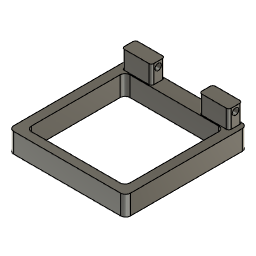
Korry_Protected_Base (Autodesk Fusion 360 design; units mm, degrees)
Autodesk Fusion 360 part; units mm, degrees
note: some values were not read from the file. Chosen so that the rebuilt part matches the saved one: which face or edge a step refers to. Set by a fixed rule: which sketch regions a step uses.
sketch "Sketch1" plane through (0, 0, 0) normal (0, 0, 1) x (1, 0, 0)
  line L0 (1, 0) -> (22.7, 0)
  line L1 (23.7, 1) -> (23.7, 23.7)
  line L2 (22.7, 24.7) -> (1, 24.7)
  line L3 (0, 23.7) -> (0, 1)
  line L4 (2.85, 21.75) -> (20.85, 21.75)
  line L5 (21.85, 20.75) -> (21.85, 2.75)
  line L6 (20.85, 1.75) -> (2.85, 1.75)
  line L7 (1.85, 2.75) -> (1.85, 20.75)
  arc A0 (2.85, 21.75) -> (1.85, 20.75) centre (2.85, 20.75) ccw
  arc A1 (1.85, 2.75) -> (2.85, 1.75) centre (2.85, 2.75) ccw
  arc A2 (21.85, 20.75) -> (20.85, 21.75) centre (20.85, 20.75) ccw
  arc A3 (20.85, 1.75) -> (21.85, 2.75) centre (20.85, 2.75) ccw
  arc A4 (1, 24.7) -> (0, 23.7) centre (1, 23.7) ccw
  arc A5 (22.7, 0) -> (23.7, 1) centre (22.7, 1) ccw
  arc A6 (0, 1) -> (1, 0) centre (1, 1) ccw
  arc A7 (23.7, 23.7) -> (22.7, 24.7) centre (22.7, 23.7) ccw
  point P0 (23.7, 0)
  point P1 (0, 24.7)
  point P2 (1.85, 21.75)
  point P3 (21.85, 21.75)
  point P4 (1.85, 1.75)
  dimension "d1" = 23.7
  dimension "d2" = 24.7
  dimension "d3" = 20
  dimension "d4" = 20
  dimension "d6" = 1.75
  dimension "d40" = 1.85
  dimension "d63" = 1
  dimension "d64" = 1
  dimension "d65" = 1
  dimension "d66" = 1
  dimension "d67" = 1
  dimension "d68" = 1
  dimension "d69" = 1
  dimension "d70" = 1
  constraint horizontal L0
  constraint vertical L1
  constraint horizontal L2
  constraint vertical L3
  constraint horizontal L4
  constraint vertical L5
  constraint horizontal L6
  constraint vertical L7
  constraint coincident P2 L4
  constraint coincident P2 L7
  constraint tangent L4 A0
  constraint tangent L7 A0
  constraint coincident P4 L6
  constraint coincident P4 L7
  constraint tangent L6 A1
  constraint tangent L7 A1
  constraint coincident P3 L4
  constraint coincident P3 L5
  constraint tangent L4 A2
  constraint tangent L5 A2
  constraint tangent L5 A3
  constraint tangent L6 A3
  constraint coincident P1 L2
  constraint coincident P1 L3
  constraint tangent L2 A4
  constraint tangent L3 A4
  constraint coincident P0 L0
  constraint coincident P0 L1
  constraint tangent L0 A5
  constraint tangent L1 A5
  constraint coincident origin L0
  constraint coincident origin L3
  constraint tangent L0 A6
  constraint tangent L3 A6
  constraint tangent L2 A7
  constraint tangent L1 A7
  measures "d1" distance of origin P0
  measures "d2" distance of origin P1
  measures "d3" distance of P2 P3
  measures "d4" distance of P2 P4
  measures "d6" distance of L0 L6
  measures "d40" distance of L3 L7
  measures "d63" radius of A0
  measures "d64" radius of A1
  measures "d65" radius of A2
  measures "d66" radius of A3
  measures "d67" radius of A4
  measures "d68" radius of A5
  measures "d69" radius of A6
  measures "d70" radius of A7
extrude "Extrude1" add sketch "Sketch1" along normal blind 4
sketch "Sketch2" plane through (0, 0, 4) normal (0, 0, 1) x (-1, 0, 0)
  line L0 (-20.85, -1.75) -> (-2.85, -1.75)
  line L1 (-1.85, -2.75) -> (-1.85, -20.75)
  line L2 (-2.85, -21.75) -> (-20.85, -21.75)
  line L3 (-21.85, -20.75) -> (-21.85, -2.75)
  line L4 (0, -23.7) -> (0, -1)
  line L5 (-1, 0) -> (-22.7, 0)
  line L6 (-23.7, -1) -> (-23.7, -23.7)
  line L7 (-22.7, -24.7) -> (-1, -24.7)
  line L8 (-1.5, -24.7) -> (-6.5, -24.7)
  line L9 (-7, -24.2) -> (-7, -22.45)
  line L10 (-6.5, -21.95) -> (-1.5, -21.95)
  line L11 (-1, -22.45) -> (-1, -24.2)
  line L12 (-22.2, -24.7) -> (-17.2, -24.7)
  line L13 (-16.7, -24.2) -> (-16.7, -22.45)
  line L14 (-17.2, -21.95) -> (-22.2, -21.95)
  line L15 (-22.7, -22.45) -> (-22.7, -24.2)
  arc A0 (-7, -24.2) -> (-6.5, -24.7) centre (-6.5, -24.2) ccw
  arc A1 (-6.5, -21.95) -> (-7, -22.45) centre (-6.5, -22.45) ccw
  arc A2 (-17.2, -24.7) -> (-16.7, -24.2) centre (-17.2, -24.2) ccw
  arc A3 (-16.7, -22.45) -> (-17.2, -21.95) centre (-17.2, -22.45) ccw
  arc A4 (-1.85, -2.75) -> (-2.85, -1.75) centre (-2.85, -2.75) ccw
  arc A5 (-2.85, -21.75) -> (-1.85, -20.75) centre (-2.85, -20.75) ccw
  arc A6 (-21.85, -20.75) -> (-20.85, -21.75) centre (-20.85, -20.75) ccw
  arc A7 (-20.85, -1.75) -> (-21.85, -2.75) centre (-20.85, -2.75) ccw
  arc A8 (0, -1) -> (-1, 0) centre (-1, -1) ccw
  arc A9 (-22.7, 0) -> (-23.7, -1) centre (-22.7, -1) ccw
  arc A10 (-1, -24.7) -> (0, -23.7) centre (-1, -23.7) ccw
  arc A11 (-23.7, -23.7) -> (-22.7, -24.7) centre (-22.7, -23.7) ccw
  arc A12 (-1, -22.45) -> (-1.5, -21.95) centre (-1.5, -22.45) ccw
  arc A13 (-1.5, -24.7) -> (-1, -24.2) centre (-1.5, -24.2) ccw
  arc A14 (-22.7, -24.2) -> (-22.2, -24.7) centre (-22.2, -24.2) ccw
  arc A15 (-22.2, -21.95) -> (-22.7, -22.45) centre (-22.2, -22.45) ccw
  point P0 (-1, -24.7)
  point P1 (-7, -24.7)
  point P2 (-22.7, -24.7)
  point P3 (-16.7, -24.7)
  dimension "d49" = 6
  dimension "d50" = 6
  dimension "d51" = 0.5
  dimension "d52" = 0.5
  dimension "d53" = 0.5
  dimension "d54" = 0.5
  dimension "d76" = 0.5
  dimension "d77" = 0.5
  dimension "d78" = 0.5
  dimension "d79" = 0.5
  constraint horizontal L8
  constraint vertical L9
  constraint horizontal L10
  constraint vertical L11
  constraint coincident P0 L7.end
  constraint horizontal L12
  constraint vertical L13
  constraint horizontal L14
  constraint vertical L15
  constraint coincident P2 L7.start
  constraint coincident P1 L8
  constraint coincident P1 L9
  constraint tangent L8 A0
  constraint tangent L9 A0
  constraint tangent L9 A1
  constraint tangent L10 A1
  constraint coincident P3 L12
  constraint coincident P3 L13
  constraint tangent L12 A2
  constraint tangent L13 A2
  constraint tangent L13 A3
  constraint tangent L14 A3
  constraint tangent L10 A12
  constraint tangent L11 A12
  constraint coincident P0 L11
  constraint coincident P0 L8
  constraint tangent L11 A13
  constraint tangent L8 A13
  constraint coincident P2 L12
  constraint coincident P2 L15
  constraint tangent L12 A14
  constraint tangent L15 A14
  constraint tangent L14 A15
  constraint tangent L15 A15
  measures "d49" distance of P0 P1
  measures "d50" distance of P2 P3
  measures "d51" radius of A0
  measures "d52" radius of A1
  measures "d53" radius of A2
  measures "d54" radius of A3
  measures "d76" radius of A12
  measures "d77" radius of A13
  measures "d78" radius of A14
  measures "d79" radius of A15
extrude "Extrude7" add sketch "Sketch2" along normal blind 5 contours L7 L8 L9 L10 L11 A0 A1 A12 A13 | L7 L12 L13 L14 L15 A2 A3 A14 A15
sketch "Sketch6" plane through (22.7, 0, 0) normal (1, 0, 0) x (0, 1, 0)
  line L0 (24.2, 9) -> (21.95, 9)
  line L1 (21.95, 9) -> (21.95, 4)
  line L2 (21.95, 4) -> (24.2, 4)
  line L3 (21.95, 4) -> (24.2, 9) construction
  line L4 (21.95, 9) -> (24.7, 4.3362) construction
  circle A0 centre (23.325, 6.6681) radius 0.65
  line L5 (24.2, 4) -> (24.2, 9)
  line L6 (22.45, 4) -> (24.2, 4)
  line L7 (24.2, 4) -> (24.2, 9)
  line L8 (24.2, 9) -> (22.45, 9)
  line L9 (22.45, 9) -> (22.45, 4)
  dimension "d57" = 1.3
  dimension "d80" = 2.3319
  constraint coincident L1.end L2.start
  constraint coincident L0.start L3.end
  constraint coincident L0.end L1.start
  constraint midpoint L4 A0.centre
  measures "d57" diameter of A0
  measures "d80" distance of L0 A0.centre
extrude "Extrude13" cut sketch "Sketch6" against normal blind 30 contours A0
extrude "Extrude12" cut 2 faces at (18.8667, 23.7833, 9) (3.1667, 23.7833, 9) along direction (0, 0, -1) blind 1.3
extrude "Extrude10" [suppressed]
extrude "Extrude8" [suppressed]
sketch "Sketch8" plane through (1, 0, 0) normal (-1, 0, 0) x (0, -1, 0)
  line L0 (-24.2, 4) -> (-22.45, 4)
  line L1 (-22.45, 9) -> (-24.2, 9)
  line L2 (-22.45, 9) -> (-24.2, 4) construction
  line L3 (-22.45, 4) -> (-24.2, 9) construction
  circle A0 centre (-23.325, 6.5) radius 0.65
  line L4 (-22.45, 4) -> (-22.45, 9)
  line L5 (-24.2, 9) -> (-24.2, 4)
  line L6 (-24.2, 4) -> (-22.45, 4)
  line L7 (-22.45, 4) -> (-22.45, 9)
  line L8 (-22.45, 9) -> (-24.2, 9)
  line L9 (-24.2, 9) -> (-24.2, 4)
  dimension "d73" = 1.3
  constraint coincident L1.start L2.start
  constraint coincident L0.start L2.end
  constraint coincident L0.end L3.start
  constraint coincident L1.end L3.end
  constraint midpoint L3 A0.centre
  measures "d73" diameter of A0
extrude "Extrude11" [suppressed]
extrude "Extrude9" [suppressed]
extrude "Extrude2" [suppressed]
sketch "Sketch4" plane through (1.5, 0, 0) normal (-1, 0, 0) x (0, -1, 0)
  line L0 (-24.3999, 4) -> (-22.3999, 4)
  line L1 (-22.3999, 4) -> (-22.3999, 8)
  line L2 (-22.3999, 8) -> (-24.3999, 8)
  line L3 (-24.3999, 8) -> (-24.3999, 4)
  circle A0 centre (-22.95, 6) radius 0.75
  point P0 (-22.95, 6)
  dimension "d34" = 1.5
  constraint coincident P0 A0.centre
  measures "d34" diameter of A0
extrude "Extrude5" [suppressed]
extrude "Extrude3" [suppressed]
sketch "Sketch5" plane through (22.4, 0, 0) normal (1, 0, 0) x (0, 1, 0)
  line L0 (22.3999, 4) -> (24.3999, 4)
  line L1 (24.3999, 4) -> (24.3999, 8)
  line L2 (24.3999, 8) -> (22.3999, 8)
  line L3 (22.3999, 8) -> (22.3999, 4)
  circle A0 centre (22.95, 6) radius 0.75
  dimension "d37" = 1.5
  measures "d37" diameter of A0
extrude "Extrude6" [suppressed]
extrude "Extrude4" [suppressed]
